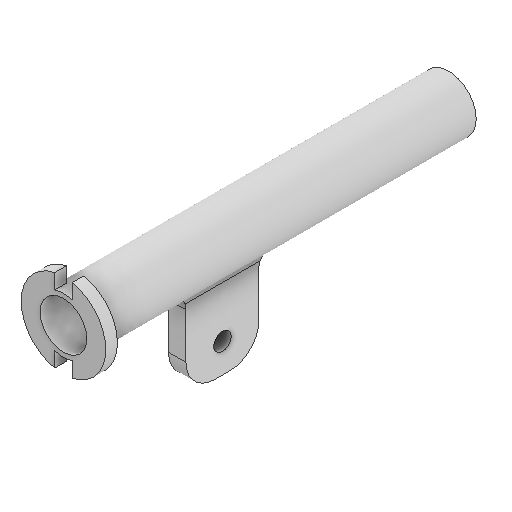
# Autodesk Inventor part: Tubo
Saved by Autodesk Inventor 2025.2 (Build 292293000, 293)
## iProperties
Created: 2025-05-03
Part Number: Tubo
Material: Genérico
Document SubType Name: Modeling
Designer: acer
Density: 1 g/cm^3
Appearance: Valor por defecto
Author: acer
Autodesk Inventor part; units mm, degrees
ref_plane "YZ Plane" through (0, 0, 0) normal (1, 0, 0) x (0, 1, 0)
ref_plane "XZ Plane" through (0, 0, 0) normal (0, 1, 0) x (-1, 0, 0)
ref_plane "XY Plane" through (0, 0, 0) normal (0, 0, 1) x (1, 0, 0)
sketch "Boceto2" plane through (0, 0, 0) normal (0, 0, 1) x (1, 0, 0)
  circle A0 centre (0, 0) radius 9.5
  circle A1 centre (0, 0) radius 5.5
  constraints: 2 centre point, 1 coincident
extrude "Extrusión1" add sketch "Boceto2" along normal blind 2
sketch "Boceto3" plane through (0, 0, 2) normal (0, 0, 1) x (1, 0, 0)
  circle A0 centre (0, 0) radius 9.5
  circle A1 centre (0, 0) radius 8
  dimension "d5" = 16
  constraints: 2 centre point, 2 coincident
  measures "d5" diameter of A1
extrude "Extrusión2" add sketch "Boceto3" along normal blind 130
sketch "Boceto4" plane through (0, 0, 132) normal (0, 0, 1) x (1, 0, 0)
  circle A0 centre (0, 0) radius 9.5
  circle A1 centre (0, 0) radius 8
  circle A2 centre (0, 0) radius 14.5
  line L0 (3, 14.186261) -> (3, -14.186261)
  line L1 (-3, 14.186261) -> (-3, -14.186261)
  point P0 (3, 0)
  point P1 (-3, 0)
  point P2 (-3, 9.013878)
  point P3 (-3, -9.013878)
  point P4 (3, -9.013878)
  point P5 (3, 9.013878)
  dimension "d36" = 19
  dimension "d37" = 5
  dimension "d38" = 3
  dimension "d39" = 3
  constraints: 4 end point, 4 point on circle, 2 midpoint, 1 centre point, 1 parallel, 1 vertical
  measures "d36" diameter of A0
  measures "d37" radial gap between concentric circles of A0 A2
  measures "d38" distance of point (3, 0) point (0, 0)
  measures "d39" distance of point (-3, 0) point (0, 0)
extrude "Extrusión3" add sketch "Boceto4" against normal blind 4 contours A0 L0 A2 | A0 L1 A2
sketch "Boceto5" plane through (0, 0, 128) normal (0, 0, -1) x (-1, 0, 0)
  line L0 (9.380832, 1.5) -> (10.897247, 1.5)
  line L1 (-9.380832, 1.5) -> (-10.897247, 1.5)
  line L2 (-9.380832, -1.5) -> (-10.897247, -1.5)
  line L3 (9.380832, -1.5) -> (10.897247, -1.5)
  arc A0 (-9.380832, 1.5) -> (-9.380832, -1.5) centre (0, 0) ccw
  arc A1 (9.380832, -1.5) -> (9.380832, 1.5) centre (0, 0) ccw
  line L4 (-10.897247, 1.5) -> (-12.409674, 1.5)
  line L5 (-10.897247, -1.5) -> (-12.409674, -1.5)
  line L6 (10.897247, 1.5) -> (12.409674, 1.5)
  line L7 (10.897247, -1.5) -> (12.409674, -1.5)
  arc A2 (-12.409674, 1.5) -> (-12.409674, -1.5) centre (0, 0) ccw
  arc A3 (12.409674, -1.5) -> (12.409674, 1.5) centre (0, 0) ccw
  constraints: 16 end point, 8 point on circle, 4 centre point, 4 point on line, 1 coincident, 1 horizontal, 1 parallel
extrude "Extrusión4" [suppressed]
sketch "Boceto6" plane through (0, 0, 128) normal (0, 0, -1) x (-1, 0, 0)
  arc A0 (-3, -9.013878) -> (3, -9.013878) centre (0, 0) ccw
  line L0 (-2.5, -20.682789) -> (-2.5, -15.634719)
  line L1 (-3, -9.013878) -> (-3, -39.013878)
  line L2 (3, -9.013878) -> (3, -39.013878)
  line L3 (-3, -39.013878) -> (3, -39.013878)
  point P0 (-1.5, -10.897247)
  point P1 (-1.5, -9.380832)
  constraints: 6 end point, 2 point on circle, 1 centre point, 1 coincident, 1 horizontal, 1 vertical, 1 other
extrude "Extrusión5" add sketch "Boceto6" along normal blind 60
sketch "Boceto7" plane through (0, 0, 128) normal (0, 0, 1) x (1, 0, 0)
  line L0 (-3, -39.013878) -> (-3, -9.013878)
  line L1 (-3, -9.013878) -> (-3, -39.013878)
  line L2 (3, -39.013878) -> (-3, -39.013878)
  line L3 (-3, -39.013878) -> (3, -39.013878)
  arc A0 (-3, -9.013878) -> (3, -9.013878) centre (0, 0) ccw
  line L4 (3, -39.013878) -> (3, -9.013878)
  circle A1 centre (0, 0) radius 9.5
  constraints: 6 end point, 1 coincident, 1 collinear, 1 horizontal, 1 perpendicular, 3 other
extrude "Extrusión6" cut sketch "Boceto7" against normal blind 35 contours L0 A0 L4 L2
fillet "Empalme1" radius 10 2 edges at (0, -39.0139, 93) (0, -39.0139, 68)
fillet "Empalme2" radius 4 4 edges at (0, -9.5, 93) (3, -9.0139, 80.5) (-3, -9.0139, 80.5) (0, -9.5, 68)
sketch "Boceto8" plane through (3, -39.013878, 83) normal (1, 0, 0) x (0, 0, -1)
  arc A0 (-10, 10) -> (0, 0) centre (0, 10) ccw projected
  circle A1 centre (2.5, 10) radius 3
  point P0 (83, 39.013878)
  point P1 (15, 10)
  constraints: 1 centre point
extrude "Extrusión7" cut sketch "Boceto8" against normal blind 6
